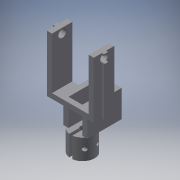
# Autodesk Inventor part: servoplace
Saved by Autodesk Inventor 2017 (Build 210142000, 142)
## iProperties
Created: 2018-08-06
Part Number: servoplace
Material: Generic
Document SubType Name: Sheet Metal
Designer: Bardo91
Density: 1 g/cm^3
Sheet Metal Rule: Default_mm
Appearance: Default
Author: Bardo91
Autodesk Inventor part; units mm, degrees
ref_plane "YZ Plane" through (0, 0, 0) normal (1, 0, 0) x (0, 1, 0)
ref_plane "XZ Plane" through (0, 0, 0) normal (0, 1, 0) x (-1, 0, 0)
ref_plane "XY Plane" through (0, 0, 0) normal (0, 0, 1) x (1, 0, 0)
sketch "Sketch1" plane through (0, 0, 0) normal (0, 0, 1) x (1, 0, 0)
  line L0 (0, 0) -> (13.5, 0)
  line L1 (13.5, 0) -> (13.5, 28.5)
  line L2 (13.5, 28.5) -> (0, 28.5)
  line L3 (0, 28.5) -> (0, 0)
  line L4 (-5, 33.5) -> (18.5, 33.5)
  line L5 (18.5, 33.5) -> (18.5, -5)
  line L6 (18.5, -5) -> (-5, -5)
  line L7 (-5, -5) -> (-5, 33.5)
  line L8 (6.75, -5) -> (-11.25, -5)
  line L9 (-11.25, -5) -> (-11.25, 15)
  line L10 (-11.25, 15) -> (-5, 15)
  line L11 (6.75, -5) -> (24.75, -5)
  line L12 (24.75, -5) -> (24.75, 15)
  line L13 (24.75, 15) -> (18.5, 15)
  dimension "d0" = 13.5
  dimension "d1" = 28.5
  dimension "d2" = 5
  dimension "d5" = 18
  dimension "d6" = 20
  dimension "d7" = 18
  dimension "d8" = 20
  constraints: 28 end point, 7 perpendicular, 6 point on line, 2 horizontal, 1 midpoint, 3 other
  measures "d0" distance of L0.start L0.end
  measures "d1" distance of L0.end L1.end
  measures "d2" distance between parallel lines of L2 L4
  measures "d5" distance of L8.start L8.end
  measures "d6" distance of L8.end L9.end
  measures "d7" distance of L8.start L11.end
  measures "d8" distance of L11.end L12.end
extrude "Extrusion1" add sketch "Sketch1" along normal blind 5
sketch "Sketch2" plane through (0, 0, 0) normal (0, 0, -1) x (-1, 0, 0)
  line L0 (11.25, 15) -> (11.25, -5) projected
  line L1 (11.25, -5) -> (11.25, 15)
  line L2 (11.25, 15) -> (16.25, 15)
  line L3 (16.25, 15) -> (16.25, -5)
  line L4 (16.25, -5) -> (11.25, -5)
  line L5 (11.25, -5) -> (-24.75, -5) projected
  line L6 (-24.75, -5) -> (-29.75, -5)
  line L7 (-29.75, -5) -> (-29.75, 15)
  line L8 (-29.75, 15) -> (-24.75, 15)
  line L9 (-24.75, -5) -> (-24.75, 15) projected
  line L10 (-24.75, 15) -> (-24.75, -5)
  line L11 (-29.75, 5) -> (-29.75, 3)
  line L12 (-29.75, 3) -> (-31.75, 3)
  line L13 (-31.75, 3) -> (-31.75, 7)
  line L14 (-31.75, 7) -> (-29.75, 7)
  line L15 (16.25, 5) -> (18.25, 5)
  line L16 (18.25, 5) -> (18.25, 3)
  line L17 (18.25, 3) -> (16.25, 3)
  line L18 (18.25, 5) -> (18.25, 7)
  line L19 (18.25, 7) -> (16.25, 7)
  point P0 (0, 0)
  dimension "d9" = 5
  dimension "d10" = 5
  dimension "d58" = 2
  dimension "d59" = 2
  dimension "d60" = 4
  dimension "d61" = 2
  dimension "d62" = 2
  dimension "d63" = 2
  constraints: 34 end point, 9 point on line, 8 perpendicular, 2 collinear, 2 midpoint, 1 horizontal
  measures "d9" distance of L0.start L2.end
  measures "d10" distance of L5.end L6.end
  measures "d58" distance of L11.start L11.end
  measures "d59" distance of L11.end L12.end
  measures "d60" distance of L12.end L13.end
  measures "d61" distance of L15.start L15.end
  measures "d62" distance of L15.end L16.end
  measures "d63" distance of L15.end L18.end
extrude "Extrusion2" add sketch "Sketch2" against normal blind 55.5
sketch "Sketch3" plane through (-16.25, -5, 0) normal (-1, 0, 0) x (0, 0, 1)
  line L0 (55.5, 20) -> (55.5, 0) projected
  line L1 (55.5, 10) -> (50.5, 10)
  circle A0 centre (50.5, 10) radius 3.75
  point P0 (0, 5)
  dimension "d13" = 5
  dimension "d14" = 7.5
  constraints: 2 end point, 1 centre point, 1 coincident, 1 horizontal, 1 midpoint
  measures "d13" distance of L1.start L1.end
  measures "d14" diameter of A0
extrude "Extrusion3" cut sketch "Sketch3" along normal through all both and the other way through all
sketch "Sketch10" plane through (0, 0, 0) normal (0, 0, -1) x (-1, 0, 0)
  line L0 (-13.5, 28.5) -> (-13.5, 0) projected
  line L1 (-13.5, 0) -> (-18.5, 0)
  line L2 (-18.5, 0) -> (-18.5, 33.5)
  line L3 (-18.5, 33.5) -> (-13.5, 33.5)
  line L4 (-13.5, 33.5) -> (-13.5, 0)
  line L5 (0, 0) -> (0, 28.5) projected
  line L6 (5, 33.5) -> (5, 15) projected
  line L7 (0, 0) -> (5, 0)
  line L8 (5, 0) -> (5, 33.5)
  line L9 (5, 33.5) -> (0, 33.5)
  line L10 (0, 33.5) -> (0, 0)
  constraints: 16 end point, 4 parallel, 2 horizontal, 2 perpendicular
extrude "Extrusion10" add sketch "Sketch10" along normal blind 21.5
sketch "Sketch11" plane through (0, 0, -21.5) normal (0, 0, -1) x (-1, 0, 0)
  line L0 (-13.5, 28.5) -> (-13.5, 0) projected
  line L1 (-13.5, 0) -> (-13.5, 7)
  line L2 (-18.5, 33.5) -> (-18.5, 0) projected
  line L3 (-6.75, 7) -> (-6.75, 13)
  line L4 (-6.75, 13) -> (-16.8526, 13)
  line L5 (-6.75, 13) -> (3.3526, 13)
  line L6 (-6.75, 13) -> (-8.25, 13)
  line L7 (-6.75, 13) -> (-5.25, 13)
  arc A0 (-16.8526, 13) -> (-8.25, -4.6539) centre (-6.75, 7) ccw
  arc A1 (-5.25, -4.6539) -> (3.3526, 13) centre (-6.75, 7) ccw
  arc A2 (-5.25, 5) -> (-6.75, 9.5) centre (-6.75, 7) ccw
  arc A3 (-8.25, 9) -> (-8.25, 5) centre (-6.75, 7) ccw
  line L8 (-5.25, 13) -> (-5.25, 9)
  line L9 (-5.25, 7) -> (-5.25, -4.6539)
  line L10 (-8.25, 13) -> (-8.25, 9)
  line L11 (-8.25, 7) -> (-8.25, -4.6539)
  line L12 (-13.5, 7) -> (-8.25, 7)
  line L13 (-5.25, 7) -> (0, 7)
  point P0 (0, 0)
  dimension "d45" = 7
  dimension "d47" = 6
  dimension "d48" = 1.5
  dimension "d49" = 1.5
  constraints: 24 end point, 9 point on circle, 7 perpendicular, 7 point on line, 4 centre point, 1 coincident, 1 tangent, 1 vertical
  measures "d45" distance of L0.end L1.end
  measures "d47" distance of L3.start L3.end
  measures "d48" distance of L3.end L6.end
  measures "d49" distance of L3.end L7.end
extrude "Extrusion11" add sketch "Sketch11" along normal blind 20 contours L4 L10 A3 L12 L0 | L0 L12 A3 L11 A0 L4 | L8 L5 A1 L9 A2
sketch "Sketch12" plane through (18.5, 15, 5) normal (1, 0, 0) x (0, 0, -1)
  line L0 (26.5, -2) -> (26.5, -6) projected
  line L1 (26.5, -10) -> (46.5, -10) projected
  line L2 (26.5, -6) -> (26.5, -10)
  line L3 (26.5, -15) -> (26.5, -8) projected
  line L4 (26.5, -10) -> (26.5, -8)
  line L5 (26.5, -8) -> (46.4389, -8)
  line L6 (36.4695, -8) -> (36.4695, -15)
  line L7 (36.4695, -8) -> (36.4695, -2)
  line L8 (36.4695, -8) -> (42.4695, -8) construction
  line L9 (36.4695, -2) -> (36.4695, -4)
  circle A0 centre (36.4695, -4) radius 1.75
  circle A1 centre (36.4695, -15) radius 1.75
  point P0 (5, -15)
  dimension "d52" = 90
  dimension "d53" = 2
  dimension "d54" = 3.5
  dimension "d55" = 3.5
  constraints: 14 end point, 3 perpendicular, 2 centre point, 2 coincident, 1 collinear, 1 horizontal, 1 midpoint, 1 point on line, 1 vertical
  measures "d52" angle of L8 L7
  measures "d53" distance of L7.end L9.end
  measures "d54" diameter of A0
  measures "d55" diameter of A1
extrude "Extrusion12" cut sketch "Sketch12" against normal through all contours A0 L7 | L7 A0 | A1
equation "\"BendRadius\" = Thickness"
equation "\"BendReliefWidth\" = Thickness"
equation "\"BendReliefDepth\" = 0.5 * Thickness"
equation "\"CornerReliefSize\" = 4 * Thickness"
equation "\"MinimumRemnant\" = 2 * Thickness"
equation "\"TransitionRadius\" = BendRadius"
equation "\"JacobiRadiusSize\" = BendRadius"
equation "\"GapSize\" = Thickness"
equation "\"Thickness\" = 0.5"
body "Solid1"
